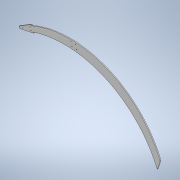
# Autodesk Inventor part: spoke
Saved by Autodesk Inventor 2020.3 (Build 243373000, 373)
## iProperties
Created: 2020-11-01
Part Number: spoke
Material: Generic
Document SubType Name: Modeling
Designer: Martijn
Density: 1 g/cm^3
Appearance: Default
Mass: 104.035 g
Surface Area: 584.811 cm^2
Volume: 104.035 cm^3
Author: Martijn
Autodesk Inventor part; units mm, degrees
ref_plane "YZ Plane" through (0, 0, 0) normal (1, 0, 0) x (0, 1, 0)
ref_plane "XZ Plane" through (0, 0, 0) normal (0, 1, 0) x (-1, 0, 0)
ref_plane "XY Plane" through (0, 0, 0) normal (0, 0, 1) x (1, 0, 0)
sketch "Sketch1" plane through (0, 0, 0) normal (0, 0, 1) x (1, 0, 0)
  arc A0 (670.9948, -199.4141) -> (0, 0) centre (254.9219, -370.8299) ccw
  arc A1 (657.7848, -239.4141) -> (30, 0) centre (229.3296, -420.1103) ccw
  arc A2 (657.7848, -239.4141) -> (670.9948, -199.4141) centre (0, 0) ccw
  line L0 (0, 0) -> (30, 0)
  line L1 (657.7848, -239.4141) -> (0, 0)
  line L2 (-143.7228, 0) -> (862.3369, 0) projected
  point P0 (0, 0)
  dimension "d1" = 30
  dimension "d2" = 40
  dimension "d4" = 20
  dimension "d5" = 465
  dimension "d6" = 450
  dimension "d22" = 700
  constraints: 6 point on circle, 4 end point, 3 centre point, 1 coincident, 1 horizontal
  measures "d1" distance of L0.start L0.end
  measures "d2" vertical distance of L1.start A0.start
  measures "d4" angle of L1 L2
  measures "d5" radius of A1
  measures "d6" radius of A0
  measures "d22" radius of A2
extrude "Extrusion1" add sketch "Sketch1" along normal blind 4 contours A2 A1 L2 A0 | L2 A1 L0 A0
sketch "Sketch2" plane through (0, 0, 4) normal (0, 0, 1) x (1, 0, 0)
  arc A0 (670.9948, -199.4141) -> (0, 0) centre (254.9219, -370.8299) ccw projected
  arc A1 (87.1309, 22.5434) -> (74.166, 50.9844) centre (0, 0) ccw
  line L0 (74.166, 50.9844) -> (0, 0)
  line L1 (0, 0) -> (87.1309, 22.5434)
  line L2 (0, 0) -> (30, 0) projected
  point P0 (78.8927, 43.3122)
  point P1 (0, 0)
  point P2 (0, 0)
  dimension "d9" = 90
  dimension "d16" = 20
  constraints: 4 end point, 2 point on circle, 1 centre point, 1 coincident, 1 tangent
  measures "d9" distance of L2.start L1.end
  measures "d16" angle of L1 L0
extrude "Extrusion2" add sketch "Sketch2" against normal blind 4
sketch "Sketch4" plane through (0, 0, 4) normal (0, 0, 1) x (1, 0, 0)
  line L0 (86.0304, 22.2587) -> (87.1309, 22.5434) projected
  line L1 (74.166, 50.9844) -> (0, 0) projected
  line L2 (87.1309, 22.5434) -> (0, 0)
  line L3 (0, 0) -> (30, 0)
  arc A0 (86.0304, 22.2587) -> (30, 0) centre (229.3296, -420.1103) ccw projected
  line L4 (30, 0) -> (86.0304, 22.2587)
  point P0 (86.0304, 22.2587)
  constraints: 6 end point, 1 horizontal
extrude "Extrusion4" cut sketch "Sketch4" against normal blind 10 contours A0 L3 L2
sketch "Sketch5" plane through (0, 0, 4) normal (0, 0, 1) x (1, 0, 0)
  line L0 (0, 0) -> (20.6017, 14.1623)
  line L1 (74.166, 50.9844) -> (0, 0) projected
  line L2 (0, 0) -> (87.1309, 22.5434) projected
  line L3 (24.203, 6.2621) -> (0, 0)
  arc A0 (24.203, 6.2621) -> (20.6017, 14.1623) centre (0, 0) ccw
  point P0 (24.203, 6.2621)
  dimension "d21" = 25
  constraints: 4 end point, 2 coincident, 2 point on circle, 1 centre point, 1 collinear, 1 point on line
  measures "d21" radius of A0
extrude "Extrusion5" cut sketch "Sketch5" against normal blind 10
sketch "Sketch6" plane through (0, 0, 4) normal (0, 0, 1) x (1, 0, 0)
  circle A0 centre (37.1637, 14.7938) radius 1.5
  circle A1 centre (71.4659, 35.9531) radius 1.5
  circle A2 centre (76.6234, 22.9969) radius 1.5
  line L0 (37.1637, 14.7938) -> (0, 0)
  line L1 (0, 0) -> (71.4659, 35.9531)
  line L2 (76.6234, 22.9969) -> (0, 0)
  line L3 (24.203, 6.2621) -> (87.1309, 22.5434) projected
  line L4 (74.166, 50.9844) -> (20.6017, 14.1623) projected
  line L5 (0, 0) -> (261.3927, 67.6302)
  line L6 (0, 0) -> (264.574, 53.8573)
  circle A3 centre (260.1726, 72.1818) radius 1.5
  circle A4 centre (264.574, 53.8573) radius 1.5
  circle A5 centre (281.2279, 70.1567) radius 1.5
  circle A6 centre (285.6292, 51.8321) radius 1.5
  line L7 (281.2279, 70.1567) -> (285.6292, 51.8321)
  line L8 (285.6292, 51.8321) -> (264.574, 53.8573)
  line L9 (264.574, 53.8573) -> (260.1726, 72.1818)
  line L10 (260.1726, 72.1818) -> (281.2279, 70.1567)
  line L11 (260.1726, 72.1818) -> (0, 0)
  dimension "d23" = 3
  dimension "d24" = 3
  dimension "d25" = 3
  dimension "d26" = 7.2
  dimension "d27" = 2.2
  dimension "d28" = 7.8
  dimension "d29" = 40
  dimension "d30" = 80
  dimension "d31" = 80
  dimension "d34" = 3
  dimension "d35" = 270
  dimension "d36" = 270
  dimension "d37" = 3
  dimension "d38" = 3
  dimension "d39" = 20
  dimension "d40" = 109
  dimension "d41" = 3
  dimension "d42" = 3
  dimension "d43" = 1
  dimension "d44" = 270
  constraints: 20 end point, 7 centre point, 2 parallel, 1 coincident, 1 collinear
  measures "d23" diameter of A1
  measures "d24" diameter of A2
  measures "d25" diameter of A0
  measures "d26" angle of L3 L0
  measures "d27" angle of L3 L2
  measures "d28" angle of L4 L1
  measures "d29" distance of L0.start L0.end
  measures "d30" distance of L0.end L1.end
  measures "d31" distance of L2.start L0.end
  measures "d34" angle of L5 L6
  measures "d35" distance of L0.end L6.end
  measures "d36" distance of L0.end L5.end
  measures "d37" diameter of A3
  measures "d38" diameter of A4
  measures "d39" distance between parallel lines of L9 L7
  measures "d40" angle of L9 L8
  measures "d41" diameter of A6
  measures "d42" diameter of A5
  measures "d43" angle of L11 L5
  measures "d44" distance of L0.end L9.end
extrude "Extrusion6" cut sketch "Sketch6" against normal blind 10 contours A0 | A2 | A1 | A4 L9 L6 | L6 L8 A4 | L11 L9 A3 | A3 L10 L11 | L9 A4 L8 | L9 L10 A3 | L8 L7 A6 | A6 L7 L8 | L10 L7 A5 | A5 L7 L10
sketch "Sketch7" plane through (0, 0, 4) normal (0, 0, 1) x (1, 0, 0)
  line L0 (20.6017, 14.1623) -> (74.166, 50.9844) projected
  arc A0 (78.8927, 43.3122) -> (74.166, 50.9844) centre (0, 0) ccw projected
  line L1 (20.6017, 14.1623) -> (74.166, 50.9844)
  line L2 (74.166, 50.9844) -> (82.5313, 50.9844)
  arc A1 (21.2689, 13.139) -> (20.6017, 14.1623) centre (0, 0) ccw
  line L3 (21.2689, 13.139) -> (82.5313, 50.9844)
  line L4 (21.2689, 13.139) -> (0, 0)
  line L5 (0, 0) -> (20.6017, 14.1623)
  point P0 (76.568, 47.3005)
  dimension "d45" = 2.8
  constraints: 10 end point, 2 point on circle, 1 centre point, 1 coincident, 1 collinear, 1 horizontal
  measures "d45" angle of L3 L0
extrude "Extrusion7" cut sketch "Sketch7" against normal blind 10 contours L0 A0 L3 A1
sketch "Sketch8" plane through (0, 0, 4) normal (0, 0, 1) x (1, 0, 0)
  line L0 (87.1309, 22.5434) -> (24.203, 6.2621) projected
  line L1 (24.203, 6.2621) -> (87.1309, 22.5434)
  arc A0 (24.48, 5.0723) -> (24.203, 6.2621) centre (0, 0) ccw
  arc A1 (88.1281, 18.2602) -> (87.1309, 22.5434) centre (0, 0) ccw
  line L2 (88.1281, 18.2602) -> (24.48, 5.0723)
  line L3 (24.48, 5.0723) -> (0, 0)
  arc A2 (24.203, 6.2621) -> (21.2689, 13.139) centre (0, 0) ccw projected
  line L4 (0, 0) -> (24.203, 6.2621)
  arc A3 (78.8927, 43.3122) -> (76.568, 47.3005) centre (0, 0) ccw projected
  dimension "d48" = 2.8
  constraints: 8 end point, 4 point on circle, 2 centre point, 2 coincident, 1 collinear, 1 concentric, 1 point on line
  measures "d48" angle of L2 L0
extrude "Extrusion8" add sketch "Sketch8" against normal blind 4 contours A1 L2 A0 L0
body "Solid1"
